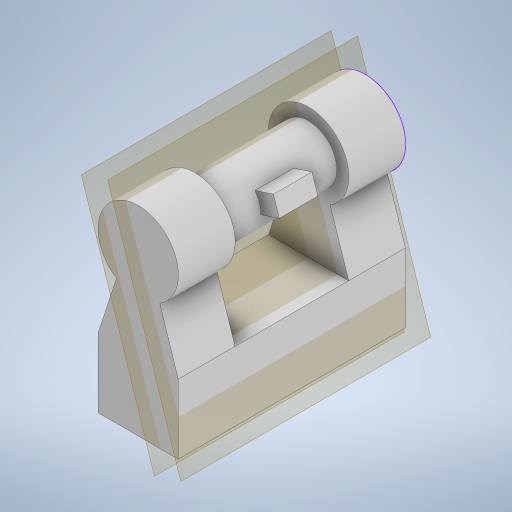
# Autodesk Inventor part: Dish antenna base
Saved by Autodesk Inventor 2024 (Build 280153000, 153)
## iProperties
Created: 2023-06-30
Part Number: Dish antenna base
Material: Generic
Document SubType Name: Modeling
Designer: hp
Density: 1 g/cm^3
Appearance: Default
Author: hp
Autodesk Inventor part; units mm, degrees
ref_plane "YZ Plane" through (0, 0, 0) normal (1, 0, 0) x (0, 1, 0)
ref_plane "XZ Plane" through (0, 0, 0) normal (0, 1, 0) x (-1, 0, 0)
ref_plane "XY Plane" through (0, 0, 0) normal (0, 0, 1) x (1, 0, 0)
sketch "Sketch1" plane through (0, 0, 0) normal (0, 0, 1) x (1, 0, 0)
  line L0 (0, 0) -> (103.82, 0)
  line L1 (0, 0) -> (0, 89.86)
  line L2 (103.82, 89.86) -> (103.82, 0)
  line L3 (103.82, 89.86) -> (80.0424, 163.0401)
  line L4 (0, 89.86) -> (23.7776, 163.0401)
  line L5 (0, 89.86) -> (103.82, 89.86)
  arc A0 (80.0424, 163.0401) -> (23.7776, 163.0401) centre (51.91, 206.88) ccw
  dimension "d1" = 89.86
  constraints: 12 end point, 2 horizontal, 2 point on circle, 1 centre point, 1 vertical
  measures "d1" distance of L0.start L1.end
sketch "Sketch2" plane through (0, 0, 0) normal (0, 0, 1) x (1, 0, 0)
  circle A0 centre (51.91, 206.8113) radius 52.09
  line L0 (0, 89.8599) -> (24.0879, 163.9947)
  line L1 (0, 89.8599) -> (77.95, 89.8599) construction
  point P0 (0, 0)
  constraints: 4 end point, 1 centre point, 1 equal length, 1 horizontal
extrude "Extrusion1" add sketch "Sketch1" along normal blind 294.64
sketch "Sketch3" plane through (103.82, 0, 0) normal (1, 0, 0) x (0, 0, -1)
  line L0 (-294.64, 89.86) -> (-294.64, 0) projected
  line L1 (0, 89.86) -> (-294.64, 89.86) projected
  line L2 (-220.98, 89.86) -> (-73.66, 89.86)
  line L3 (-73.66, 89.86) -> (-73.66, 276.7764)
  line L4 (-73.66, 276.7764) -> (-220.98, 276.7764)
  line L5 (0, 163.0401) -> (-294.64, 163.0401) projected
  line L6 (-220.98, 276.7764) -> (-220.98, 89.86)
  point P0 (0, 0)
  constraints: 8 end point, 2 perpendicular, 1 parallel, 1 point on line
extrude "Extrusion2" cut sketch "Sketch3" along normal mid plane 294.64
sketch "Sketch4" plane through (0, 0, 0) normal (0, 0, -1) x (-1, 0, 0)
  point P0 (0, 0)
sketch "Sketch5" plane through (0, 0, 0) normal (0, 0, -1) x (-1, 0, 0)
  point P0 (0, 0)
sketch "Sketch6" plane through (0, 0, 294.64) normal (0, 0, 1) x (1, 0, 0)
  point P0 (0, 0)
sketch "Sketch7" plane through (51.91, 206.88, 73.66) normal (0, 0, 1) x (1, 0, 0)
  circle A0 centre (0, 0) radius 36.83
  point P0 (-51.91, -206.88)
  dimension "d23" = 73.66
  constraints: 1 centre point
  measures "d23" diameter of A0
extrude "Extrusion3" cut sketch "Sketch7" against normal blind 30
sketch "Sketch8" plane through (51.91, 206.88, 220.98) normal (0, 0, -1) x (-1, 0, 0)
  circle A0 centre (0, 0) radius 36.83
  point P0 (51.91, -206.88)
  dimension "d26" = 73.66
  constraints: 1 centre point
  measures "d26" diameter of A0
extrude "Extrusion4" cut sketch "Sketch8" against normal blind 30
sketch "Sketch9" plane through (51.91, 206.88, 250.98) normal (0, 0, -1) x (-1, 0, 0)
  circle A0 centre (0, 0) radius 36.83
  point P0 (51.91, -206.88)
  dimension "d29" = 73.66
  constraints: 1 centre point
  measures "d29" diameter of A0
extrude "Extrusion5" add sketch "Sketch9" along normal blind 207.32
ref_plane "Work Plane2" through (86.148, 100.9846, 220.98) normal (0.9511, 0.309, 0) x (0, 0, -1)
ref_plane "Work Plane1" through (51.91, 89.86, 220.98) normal (0.9511, 0.309, 0) x (0, 0, -1)
sketch "Sketch10" plane through (86.148, 100.9846, 220.98) normal (0.9511, 0.309, 0) x (0, 0, -1)
  line L0 (0, 148.1226) -> (0, 74.4626) construction
  line L1 (0, 111.2926) -> (147.32, 111.2926) construction
  line L2 (147.32, 74.4626) -> (147.32, 148.1226) construction
  line L3 (0, 148.1226) -> (147.32, 148.1226) construction
  line L4 (73.66, 148.1226) -> (73.66, 74.4626) construction
  line L5 (0, 74.4626) -> (147.32, 74.4626) construction
  line L6 (73.66, 111.2926) -> (48.66, 111.2926) construction
  line L7 (48.66, 111.2926) -> (48.66, 123.5771) construction
  line L8 (48.66, 123.5771) -> (98.66, 123.5771)
  line L9 (98.66, 123.5771) -> (98.66, 99.0081)
  line L10 (98.66, 99.0081) -> (48.66, 99.0081)
  line L11 (48.66, 99.0081) -> (48.66, 123.5771)
  point P0 (220.98, -69.4209)
  dimension "d33" = 25
  dimension "d34" = 12.2845
  dimension "d35" = 50
  dimension "d36" = 24.569
  constraints: 16 end point, 5 midpoint, 2 parallel, 1 horizontal, 1 perpendicular, 1 point on line, 1 vertical
  measures "d33" distance of L6.start L6.end
  measures "d34" distance of L6.end L7.end
  measures "d35" distance of L9.end L10.end
  measures "d36" distance of L8.end L9.end
extrude "Extrusion6" add sketch "Sketch10" along normal blind 60
body "Solid1"
